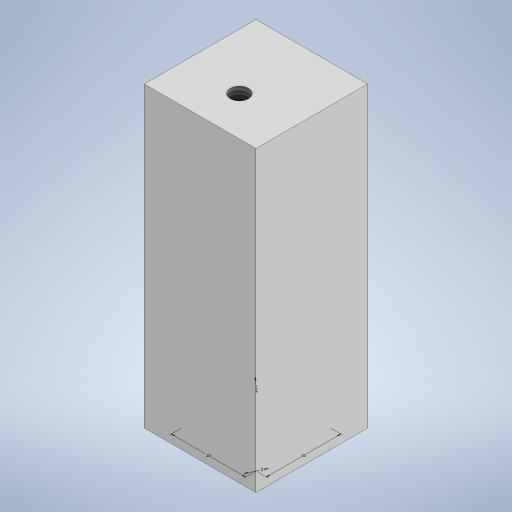
# Autodesk Inventor part: TallTower
Saved by Autodesk Inventor 2024 (Build 280153000, 153)
## iProperties
Created: 2026-03-14
Part Number: TallTower
Material: Generic
Document SubType Name: Modeling
Designer: Nathan
Density: 1 g/cm^3
Appearance: Default
Author: Nathan
Autodesk Inventor part; units mm, degrees
ref_plane "YZ Plane" through (0, 0, 0) normal (1, 0, 0) x (0, 1, 0)
ref_plane "XZ Plane" through (0, 0, 0) normal (0, 1, 0) x (-1, 0, 0)
ref_plane "XY Plane" through (0, 0, 0) normal (0, 0, 1) x (1, 0, 0)
sketch "Sketch1" plane through (0, 0, 0) normal (0, 1, 0) x (-1, 0, 0)
  line L0 (15, 15) -> (-15, 15)
  line L1 (-15, 15) -> (-15, -15)
  line L2 (-15, -15) -> (15, -15)
  line L3 (15, -15) -> (15, 15)
  line L4 (15, 15) -> (-15, -15) construction
  line L5 (-15, 15) -> (15, -15) construction
  point P0 (0, 0)
  dimension "d0" = 30
  dimension "d1" = 30
  constraints: 12 end point, 2 midpoint, 2 parallel, 1 horizontal, 1 perpendicular
  measures "d0" distance of L2.end L1.end
  measures "d1" distance of L1.end L0.end
extrude "Extrusion1" add sketch "Sketch1" along normal blind 80
sketch "Sketch2" plane through (0, 80, 0) normal (0, 1, 0) x (1, 0, 0)
  line L0 (-15, -15) -> (15, -15) construction
  line L1 (0, -15) -> (0, 3.55) construction
  line L2 (0, 3.55) -> (0, -4.45) construction
  point P0 (0, 0)
  dimension "d4" = 18.55
  dimension "d5" = 8
  constraints: 4 end point, 1 midpoint, 1 point on line, 1 vertical
  measures "d4" distance of L1.start L1.end
  measures "d5" distance of L1.end L2.end
hole "Hole1" at (0, 80, 4.45) direction (0, -1, 0) diameter 4.917 depth 21 thread size "M6x1" class "6H" standard "ISO Metric profile"
sketch "Sketch3" plane through (0, 0, 0) normal (0, -1, 0) x (1, 0, 0)
  line L0 (-10, -10) -> (10, -10) construction
  line L1 (10, -10) -> (10, 10) construction
  line L2 (10, 10) -> (-10, 10) construction
  line L3 (-10, 10) -> (-10, -10) construction
  line L4 (-10, -10) -> (10, 10) construction
  line L5 (10, -10) -> (-10, 10) construction
  circle A0 centre (10, 10) radius 2.5
  circle A1 centre (-10, -10) radius 2.5
  point P0 (0, 0)
  dimension "d20" = 20
  dimension "d21" = 20
  dimension "d22" = 5
  dimension "d23" = 5
  constraints: 12 end point, 2 centre point, 2 coincident, 2 midpoint, 2 parallel, 1 horizontal, 1 perpendicular
  measures "d20" distance of L2.end L1.end
  measures "d21" distance of L1.end L0.end
  measures "d22" diameter of A0
  measures "d23" diameter of A1
hole "Hole2" at (0, 0, 0) direction (0, 1, 0) diameter 4.917 depth 13 thread size "M6x1" class "6H" standard "ISO Metric profile"
extrude "Extrusion2" cut sketch "Sketch3" against normal blind 11
sketch "Sketch7" plane through (0, 0, 0) normal (0, -1, 0) x (1, 0, 0)
  point P0 (0, 0)
body "Solid1"
